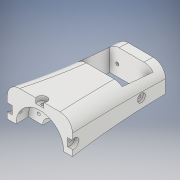
# Autodesk Inventor part: AA008
Saved by Autodesk Inventor 2017 SP1 (Build 210196100, 196)
## iProperties
Created: 2017-09-28
Part Number: AA008
Material: ABS Plastic
Document SubType Name: Modeling
Designer: Zach
Density: 1.06 g/cm^3
Appearance: CR White
Author: Zach
Autodesk Inventor part; units mm, degrees
ref_plane "XY Plane" through (0, 0, 0) normal (0, 0, 1) x (1, 0, 0)
sketch "Sketch1" plane through (0, 0, 0) normal (0, 0, 1) x (1, 0, 0)
  line L0 (0, 0) -> (80, 0)
  line L1 (80, 0) -> (80, 82.6)
  line L2 (80, 82.6) -> (0, 82.6)
  line L3 (0, 82.6) -> (0, 0)
  dimension "d0" = 80
  dimension "d1" = 82.6
  constraints: 8 end point, 2 parallel, 1 horizontal, 1 perpendicular
  measures "d0" distance of L2.end L1.end
  measures "d1" distance of L1.end L0.end
extrude "Extrusion1" add sketch "Sketch1" along normal blind 162.5
sketch "Sketch2" plane through (0, 82.6, 0) normal (0, 1, 0) x (1, 0, 0)
  line L0 (0, -162.5) -> (80, -162.5) projected
  line L1 (-12.5, -162.5) -> (0, -162.5)
  line L2 (80, -162.5) -> (92.5, -162.5)
  line L3 (0, 0) -> (80, 0) projected
  line L4 (0, 0) -> (0, -162.5) projected
  line L5 (80, 0) -> (80, -162.5) projected
  arc A0 (-12.5, -162.5) -> (0, 0) centre (-1199.9534, 10.5733) ccw
  arc A1 (80, 0) -> (92.5, -162.5) centre (1279.9534, 10.5733) ccw
  dimension "d4" = 12.5
  dimension "d5" = 12.5
  dimension "d19" = 1200
  dimension "d20" = 1200
  constraints: 4 end point, 4 point on circle, 2 centre point, 1 collinear, 1 parallel
  measures "d4" distance of L1.start L0.start
  measures "d5" distance of L0.end L2.end
  measures "d19" radius of A0
  measures "d20" radius of A1
extrude "Extrusion2" add sketch "Sketch2" against normal blind 82.6 contours L1 A0 L4 | L5 A1 L2
sketch "Sketch4" plane through (0, 0, 0) normal (0, 0, -1) x (-1, 0, 0)
  circle A0 centre (-17.4, 59.41) radius 2.5
  circle A1 centre (-62.6, 59.41) radius 2.5
  circle A2 centre (-62.6, 23.19) radius 2.5
  circle A3 centre (-17.4, 23.19) radius 2.5
  line L0 (-80, 82.6) -> (0, 82.6) projected
  line L1 (-17.4, 23.19) -> (-62.6, 23.19) construction
  line L2 (-62.6, 23.19) -> (-62.6, 59.41) construction
  line L3 (-80, 0) -> (-80, 82.6) projected
  point P0 (0, 0)
  point P1 (-60.8187, 82.6)
  point P2 (-19.1813, 82.6)
  point P3 (-40, 23.19)
  point P4 (-40, 82.6)
  dimension "d10" = 5
  dimension "d11" = 5
  dimension "d12" = 5
  dimension "d13" = 5
  dimension "d14" = 23.19
  dimension "d15" = 45.2
  dimension "d16" = 36.22
  constraints: 4 centre point, 4 end point, 3 vertical alignment, 2 horizontal alignment, 2 midpoint, 1 horizontal, 1 perpendicular
  measures "d10" diameter of A0
  measures "d11" diameter of A1
  measures "d12" diameter of A2
  measures "d13" diameter of A3
  measures "d14" distance from line of L0 A0.centre
  measures "d15" distance of L2.end A0.centre
  measures "d16" distance of L2.end L1.end
extrude "Extrusion3" cut sketch "Sketch4" against normal blind 25
sketch "Sketch5" plane through (0, 0, 0) normal (0, 0, -1) x (-1, 0, 0)
  line L0 (12.5, 0) -> (-92.5, 0)
  line L1 (-92.5, 0) -> (-92.5, 41.3)
  line L2 (-92.5, 41.3) -> (12.5, 41.3)
  line L3 (12.5, 41.3) -> (12.5, 0)
  point P0 (0, 0)
  point P1 (12.5, 20)
  point P2 (-92.5, 20)
  dimension "d22" = 41.3
  constraints: 8 end point, 2 parallel, 2 point on line, 1 horizontal, 1 horizontal alignment, 1 perpendicular
  measures "d22" distance of L0.end L1.end
extrude "Extrusion4" cut sketch "Sketch5" against normal through all
sketch "Sketch6" plane through (0, 41.3, 0) normal (0, -1, 0) x (1, 0, 0)
  line L0 (75, 15) -> (5, 15)
  line L1 (5, 15) -> (5, 65)
  line L2 (5, 65) -> (75, 65)
  line L3 (75, 65) -> (75, 15)
  line L4 (80, 0) -> (0, 0) projected
  point P0 (40, 15)
  point P1 (40, 0)
  dimension "d25" = 70
  dimension "d26" = 50
  dimension "d27" = 15
  constraints: 8 end point, 2 midpoint, 2 parallel, 1 horizontal, 1 perpendicular, 1 vertical alignment
  measures "d25" distance of L1.end L2.end
  measures "d26" distance of L0.end L1.end
  measures "d27" distance between parallel lines of L4 L0
extrude "Extrusion5" cut sketch "Sketch6" against normal blind 32.5
sketch "Sketch8" plane through (0, 0, 0) normal (1, 0, 0) x (0, 1, 0)
  line L0 (82.6, 162.5) -> (93.8, 162.5)
  line L1 (41.3, 162.5) -> (41.3, 0) projected
  line L2 (82.6, 0) -> (41.3, 0) projected
  arc A0 (93.8, 162.5) -> (82.6, 0) centre (2580.9593, -90.5586) ccw
  line L3 (82.6, 162.5) -> (41.3, 162.5) projected
  line L4 (82.6, 162.5) -> (82.6, 0)
  point P0 (0, 0)
  dimension "d32" = 2500
  dimension "d38" = 11.2
  constraints: 4 end point, 2 point on circle, 1 centre point, 1 horizontal, 1 perpendicular
  measures "d32" radius of A0
  measures "d38" distance of L0.start L0.end
extrude "Extrusion6" add sketch "Sketch8" along normal blind 93 and the other way blind 13 contours L0 A0 L4
sketch "Sketch13" plane through (-13, 82.6, 0) normal (0, -1, 0) x (1, 0, 0)
  arc A0 (13, 0) -> (0.5, 162.5) centre (-1186.9534, -10.5733) ccw projected
  line L0 (0, 162.5) -> (0.5, 162.5) projected
  line L1 (0, 0) -> (0, 162.5) projected
  line L2 (13, 0) -> (0, 0) projected
  arc A1 (105.5, 162.5) -> (93, 0) centre (1292.9534, -10.5733) ccw projected
  line L3 (106, 0) -> (93, 0) projected
  line L4 (106, 162.5) -> (106, 0) projected
  line L5 (105.5, 162.5) -> (106, 162.5) projected
  point P0 (13, 0)
extrude "Extrusion9" cut sketch "Sketch13" against normal through all
fillet "Fillet4" radius 20 2 edges at (-3.5176, 86.9111, 81.8462) (83.5176, 86.9111, 81.8462)
sketch "Sketch15" plane through (0, 0, 162.5) normal (0, 0, 1) x (1, 0, 0)
  line L0 (80, 41.3) -> (0, 41.3) projected
  circle A0 centre (40, 41.3) radius 38.5
  point P0 (0, 0)
  dimension "d54" = 77
  constraints: 1 centre point, 1 midpoint
  measures "d54" diameter of A0
extrude "Extrusion11" cut sketch "Sketch15" against normal blind 20
sketch "Sketch17" plane through (0, 0, 142.5) normal (0, 0, 1) x (1, 0, 0)
  line L0 (75, 41.3) -> (5, 41.3) projected
  circle A0 centre (40, 41.3) radius 15.5
  point P0 (0, 0)
  dimension "d57" = 31
  constraints: 1 centre point, 1 midpoint
  measures "d57" diameter of A0
extrude "Extrusion12" cut sketch "Sketch17" against normal blind 25
sketch "Sketch18" plane through (0, 0, 142.5) normal (0, 0, 1) x (1, 0, 0)
  circle A0 centre (40, 66.3) radius 2.5
  line L0 (55.5, 41.3) -> (24.5, 41.3) projected
  circle A1 centre (18.3494, 53.8) radius 2.5
  circle A2 centre (18.3494, 28.8) radius 2.5
  circle A3 centre (40, 16.3) radius 2.5
  circle A4 centre (61.6506, 28.8) radius 2.5
  circle A5 centre (61.6506, 53.8) radius 2.5
  point P0 (0, 0)
  point P1 (40, 41.3)
  dimension "d60" = 5
  dimension "d61" = 25
  dimension "d64" = 360
  constraints: 6 centre point, 1 midpoint, 1 vertical alignment, 13 other
  measures "d60" diameter of A0
  measures "d61" distance of point (40, 41.3) A0.centre
extrude "Extrusion13" cut sketch "Sketch18" against normal blind 25
ref_plane "Work Plane3" through (0, 0, 112.5) normal (0, 0, 1) x (1, 0, 0)
sketch "Sketch20" plane through (0, 0, 112.5) normal (0, 0, 1) x (1, 0, 0)
  line L0 (55.5, 41.3) -> (24.5, 41.3) construction
  arc A0 (55.5, 41.3) -> (24.5, 41.3) centre (40, 41.3) ccw construction
  circle A1 centre (40, 41.3) radius 14
  point P0 (0, 0)
  dimension "d70" = 28
  constraints: 1 centre point, 1 coincident
  measures "d70" diameter of A1
extrude "Extrusion14" cut sketch "Sketch20" against normal blind 70
sketch "Sketch21" plane through (0, 0, 117.5) normal (0, 0, 1) x (1, 0, 0)
  line L0 (75, 41.3) -> (5, 41.3) projected
  circle A0 centre (40, 41.3) radius 2.5
  circle A1 centre (40, 49.8) radius 2
  line L1 (55.5, 41.3) -> (24.5, 41.3) projected
  point P0 (0, 0)
  dimension "d74" = 5
  dimension "d75" = 4
  dimension "d76" = 8.5
  constraints: 2 centre point, 2 midpoint, 1 vertical alignment
  measures "d74" diameter of A0
  measures "d75" diameter of A1
  measures "d76" distance of A1.centre A0.centre
extrude "Extrusion15" cut sketch "Sketch21" against normal blind 8
sketch "Sketch22" plane through (0, 0, 112.5) normal (0, 0, -1) x (-1, 0, 0)
  arc A0 (-37.5, 41.3) -> (-42.5, 41.3) centre (-40, 41.3) ccw projected
  circle A1 centre (-40, 41.3) radius 4
  point P0 (0, 0)
  dimension "d80" = 8
  constraints: 1 centre point, 1 coincident
  measures "d80" diameter of A1
extrude "Extrusion16" cut sketch "Sketch22" against normal blind 3
sketch "Sketch23" plane through (0, 0, 117.5) normal (0, 0, 1) x (1, 0, 0)
  circle A0 centre (40, 49.8) radius 2 projected
  circle A1 centre (40, 49.8) radius 4.5
  point P0 (0, 0)
  dimension "d83" = 9
  constraints: 1 centre point, 1 coincident
  measures "d83" diameter of A1
extrude "Extrusion17" cut sketch "Sketch23" against normal blind 3
sketch "Sketch25" plane through (0, 73.8, 0) normal (0, -1, 0) x (1, 0, 0)
  line L0 (75, 15) -> (5, 15) projected
  line L1 (75, 65) -> (75, 15) projected
  line L2 (5, 65) -> (75, 65) projected
  line L3 (5, 15) -> (5, 65) projected
  point P0 (0, 0)
extrude "Extrusion18" cut sketch "Sketch25" against normal through all
ref_plane "Work Plane5" through (72.5841, 93.8, 162.5) normal (0, 1, 0) x (-1, 0, 0)
sketch "Sketch27" plane through (72.5841, 93.8, 162.5) normal (0, 1, 0) x (-1, 0, 0)
  line L0 (65.1681, 0) -> (0, 0)
  line L1 (-4.9159, 0) -> (70.0841, 0)
  circle A0 centre (32.5841, -4) radius 7.5
  point P0 (72.5841, -162.5)
  point P1 (32.5841, 0)
  dimension "d91" = 15
  dimension "d94" = 4
  constraints: 4 end point, 1 centre point, 1 midpoint, 1 vertical alignment
  measures "d91" diameter of A0
  measures "d94" distance of point (32.584, 0) A0.centre
extrude "Extrusion19" cut sketch "Sketch27" against normal blind 8
sketch "Sketch29" plane through (72.5841, 85.8, 162.5) normal (0, 1, 0) x (1, 0, 0)
  circle A0 centre (-32.5841, 4) radius 2
  arc A1 (-26.2398, 0) -> (-38.9284, 0) centre (-32.5841, 4) ccw projected
  point P0 (-72.5841, 162.5)
  dimension "d95" = 4
  constraints: 1 centre point, 1 concentric, 1 horizontal alignment
  measures "d95" diameter of A0
extrude "Extrusion20" cut sketch "Sketch29" against normal through all
ref_plane "Work Plane6" through (-12.5, 41.3, 162.5) normal (1, 0, 0) x (0, 1, 0)
sketch "Sketch30" plane through (-12.5, 41.3, 162.5) normal (1, 0, 0) x (0, 1, 0)
  line L0 (32.6904, 0) -> (0, 0) projected
  circle A0 centre (16.3452, -4) radius 7.5
  point P0 (-41.3, -162.5)
  point P1 (16.3452, 0)
  dimension "d98" = 15
  dimension "d99" = 4
  constraints: 1 centre point, 1 midpoint, 1 vertical alignment
  measures "d98" diameter of A0
  measures "d99" distance from line of L0 A0.centre
extrude "Extrusion21" cut sketch "Sketch30" along normal blind 8
sketch "Sketch32" plane through (-4.5, 41.3, 162.5) normal (-1, 0, 0) x (0, 0, 1)
  circle A0 centre (-4, 16.3452) radius 2
  arc A1 (0, 22.6895) -> (0, 10.0009) centre (-4, 16.3452) ccw projected
  point P0 (-162.5, -41.3)
  dimension "d102" = 4
  constraints: 1 centre point, 1 concentric, 1 vertical alignment
  measures "d102" diameter of A0
extrude "Extrusion22" cut sketch "Sketch32" against normal through all
ref_plane "Work Plane7" through (92.5, 41.3, 162.5) normal (1, 0, 0) x (0, 1, 0)
sketch "Sketch33" plane through (92.5, 41.3, 162.5) normal (1, 0, 0) x (0, 1, 0)
  spline S0 degree 7 poles (16.3452, -2) (16.5842, -2) (16.823, -2.0333) (17.0589, -2.0999) (17.2885, -2.2007) (17.5074, -2.3374) (17.7098, -2.5118) (18.0398, -2.9108) (18.1792, -3.1324) (18.2884, -3.3855) (18.3565, -3.661) (18.3776, -3.9466) (18.3512, -4.2293) (18.2119, -4.7719) (18.0994, -5.0216) (17.9544, -5.2419) (17.785, -5.431) (17.5982, -5.5882) (17.4002, -5.7139) (16.9472, -5.9271) (16.6861, -6.0009) (16.4192, -6.0336) (16.1506, -6.0259) (15.8845, -5.9774) (15.6259, -5.8869) (15.1979, -5.6516) (15.02, -5.5245) (14.853, -5.3705) (14.7022, -5.1893) (14.5734, -4.9818) (14.4729, -4.75) (14.3444, -4.2496) (14.3167, -3.9882) (14.3298, -3.7231) (14.3837, -3.465) (14.4743, -3.2243) (14.5929, -3.0092) (14.9036, -2.5816) (15.1129, -2.383) (15.3429, -2.2275) (15.586, -2.1131) (15.8367, -2.0377) (16.0909, -2) (16.3452, -2) knots 0 0 0 0 0 0 0 0 0.152749 0.152749 0.152749 0.152749 0.152749 0.152749 0.285714 0.285714 0.285714 0.285714 0.285714 0.285714 0.421907 0.421907 0.421907 0.421907 0.421907 0.421907 0.58891 0.58891 0.58891 0.58891 0.58891 0.58891 0.71461 0.71461 0.71461 0.71461 0.71461 0.71461 0.837939 0.837939 0.837939 0.837939 0.837939 0.837939 1 1 1 1 1 1 1 1 projected
  circle A0 centre (16.3452, -4) radius 2 projected
  circle A1 centre (16.3452, -4) radius 7.5
  point P0 (-41.3, -162.5)
  dimension "d105" = 15
  constraints: 1 centre point, 1 coincident, 1 vertical alignment, 1 other
  measures "d105" diameter of A1
extrude "Extrusion23" cut sketch "Sketch33" against normal blind 8
sketch "Sketch34" plane through (75, 41.3, 15) normal (-1, 0, 0) x (0, 0, 1)
  line L0 (50, 0) -> (0, 0) projected
  line L1 (50, 0) -> (50, 40.0121) projected
  line L2 (0, 0) -> (0, 35.3757) projected
  circle A0 centre (25, 15) radius 2.5
  point P0 (-15, -41.3)
  point P1 (25, 0)
  dimension "d108" = 5
  dimension "d109" = 15
  constraints: 1 centre point, 1 midpoint, 1 vertical alignment, 1 other
  measures "d108" diameter of A0
  measures "d109" distance from line of L0 A0.centre
extrude "Extrusion24" cut sketch "Sketch34" along normal through all both and the other way through all
ref_plane "Work Plane8" through (92.5, 41.3, 162.5) normal (1, 0, 0) x (0, 1, 0)
ref_plane "Work Plane9" through (-12.5, 41.3, 162.5) normal (1, 0, 0) x (0, 1, 0)
sketch "Sketch36" plane through (92.5, 41.3, 162.5) normal (1, 0, 0) x (0, 1, 0)
  spline S0 degree 8 poles (15, -120) (15.2604, -120) (15.5204, -120.031) (15.7781, -120.0928) (16.0315, -120.1862) (16.2777, -120.3125) (16.5128, -120.4735) (16.7315, -120.671) (17.0917, -121.1064) (17.246, -121.3412) (17.3756, -121.6073) (17.4705, -121.8984) (17.5239, -122.2056) (17.5327, -122.5187) (17.4971, -122.8272) (17.3432, -123.4264) (17.2249, -123.7056) (17.0748, -123.9561) (16.9001, -124.1766) (16.7067, -124.3668) (16.5001, -124.5271) (16.2847, -124.6584) (15.7907, -124.8909) (15.5066, -124.9783) (15.2169, -125.0266) (14.9248, -125.0369) (14.6332, -125.0096) (14.345, -124.9439) (14.064, -124.8383) (13.5967, -124.5814) (13.4029, -124.448) (13.2178, -124.2895) (13.0453, -124.1054) (12.8898, -123.8956) (12.7564, -123.6606) (12.6504, -123.4018) (12.5087, -122.8499) (12.4728, -122.5649) (12.4746, -122.2747) (12.5151, -121.9881) (12.5922, -121.7135) (12.7006, -121.4588) (12.8326, -121.2299) (13.1724, -120.7622) (13.398, -120.5372) (13.6442, -120.3542) (13.904, -120.2108) (14.1727, -120.105) (14.4466, -120.035) (14.7232, -120) (15, -120) knots 0 0 0 0 0 0 0 0 0 0.154457 0.154457 0.154457 0.154457 0.154457 0.154457 0.154457 0.285677 0.285677 0.285677 0.285677 0.285677 0.285677 0.285677 0.421425 0.421425 0.421425 0.421425 0.421425 0.421425 0.421425 0.590168 0.590168 0.590168 0.590168 0.590168 0.590168 0.590168 0.71522 0.71522 0.71522 0.71522 0.71522 0.71522 0.71522 0.83662 0.83662 0.83662 0.83662 0.83662 0.83662 0.83662 1 1 1 1 1 1 1 1 1 projected
  circle A0 centre (15, -122.5) radius 6.5
  circle A1 centre (15, -122.5) radius 2.5 projected
  point P0 (-41.3, -162.5)
  dimension "d112" = 13
  constraints: 1 centre point, 1 vertical alignment, 2 other
  measures "d112" diameter of A0
extrude "Extrusion25" cut sketch "Sketch36" against normal blind 15
sketch "Sketch37" plane through (-12.5, 41.3, 162.5) normal (1, 0, 0) x (0, 1, 0)
  circle A0 centre (15, -122.5) radius 6.5 projected
  point P0 (-41.3, -162.5)
  constraints: 1 other
extrude "Extrusion26" cut sketch "Sketch37" along normal blind 15
equation "\"d5\" = d4"
body "Solid1"
